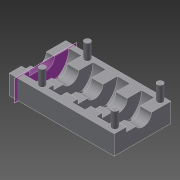
# Autodesk Inventor part: lock housing front
Saved by Autodesk Inventor 2017 (Build 210142000, 142)
## iProperties
Created: 2018-04-20
Part Number: lock housing front
Material: Generic
Document SubType Name: Modeling
Designer: natha
Density: 1 g/cm^3
Appearance: Default
Author: natha
Autodesk Inventor part; units mm, degrees
ref_plane "YZ Plane" through (0, 0, 0) normal (1, 0, 0) x (0, 1, 0)
ref_plane "XZ Plane" through (0, 0, 0) normal (0, 1, 0) x (-1, 0, 0)
sketch "Sketch1" plane through (0, 0, 0) normal (0, 0, 1) x (1, 0, 0)
  arc A0 (-18.2373, -76.3503) -> (26.9537, -71.5105) centre (0, -33.2365) ccw projected
  line L0 (26.9537, -71.5105) -> (46.8123, -71.5105) projected
  line L1 (46.8123, -71.5105) -> (46.8123, -74.3095) projected
  arc A1 (23.0377, -99.6575) -> (46.8123, -74.3095) centre (21.4123, -74.3095) ccw projected
  line L2 (23.0377, -99.6575) -> (23.0377, -92.0895) projected
  line L3 (23.0377, -92.0895) -> (-18.2373, -92.0895) projected
  line L4 (-18.2373, -76.3503) -> (-18.2373, -92.0895) projected
  arc A2 (21.4123, -99.7095) -> (46.8123, -74.3095) centre (21.4123, -74.3095) ccw projected
  line L5 (46.8123, -74.3095) -> (46.8123, -71.5105) projected
  line L6 (46.8123, -71.5105) -> (26.9537, -71.5105) projected
  arc A3 (-26.9537, -71.5105) -> (26.9537, -71.5105) centre (0, -33.2365) ccw projected
  line L7 (-26.9537, -71.5105) -> (-46.8123, -71.5105) projected
  line L8 (-46.8123, -71.5105) -> (-46.8123, -74.3095) projected
  arc A4 (-46.8123, -74.3095) -> (-21.4123, -99.7095) centre (-21.4123, -74.3095) ccw projected
  line L9 (-21.4123, -99.7095) -> (21.4123, -99.7095) projected
  line L10 (-18.2373, -92.0895) -> (-18.2373, -99.7095)
  line L11 (-18.2373, -92.0895) -> (23.0377, -92.0895)
  line L12 (23.0377, -92.0895) -> (23.0377, -99.6575)
  point P0 (0, 0)
  constraints: 6 end point, 2 collinear, 1 perpendicular, 1 point on line
ref_plane "Work Plane1" through (-46.8123, -99.7095, 22.225) normal (0, 0, -1) x (0, 1, 0)
extrude "Extrusion1" add sketch "Sketch1" along normal up to surface (22.225 mm away) contours L3 L2 A2 L9 L10
sketch "Sketch2" plane through (-18.2373, -92.0895, 22.225) normal (0, 1, 0) x (1, 0, 0)
  circle A0 centre (39.0525, 2.4765) radius 1.27 projected
  circle A1 centre (39.0525, 20.2565) radius 1.27 projected
  circle A2 centre (10.4775, 20.2565) radius 1.27 projected
  circle A3 centre (10.4775, 2.4765) radius 1.27 projected
  circle A4 centre (39.0525, 2.4765) radius 1.143
  circle A5 centre (39.0525, 20.2565) radius 1.143
  circle A6 centre (10.4775, 2.4765) radius 1.143
  circle A7 centre (10.4775, 20.2565) radius 1.143
  point P0 (18.2373, 22.225)
  dimension "d4" = 0.127
  dimension "d5" = 0.127
  dimension "d6" = 0.127
  dimension "d7" = 0.127
  constraints: 4 centre point
  measures "d4" radial gap between concentric circles of A0 A4
  measures "d5" radial gap between concentric circles of A1 A5
  measures "d6" radial gap between concentric circles of A3 A6
  measures "d7" radial gap between concentric circles of A2 A7
extrude "Extrusion2" add sketch "Sketch2" along normal blind 6.096 contours A4 | A5 | A6 | A7
ref_plane "Work Plane2" through (-15.0623, -99.7095, 0) normal (-1, 0, 0) x (0, 0, 1)
sketch "Sketch3" plane through (-15.0623, -99.7095, 0) normal (-1, 0, 0) x (0, 0, 1)
  arc A0 (8.8042, -0.8832) -> (13.0521, -0.8802) centre (10.922, 7.62) ccw projected
  circle A1 centre (10.922, 7.62) radius 3.175 projected
  line L0 (13.744, 9.3345) -> (17.399, 9.3345) projected
  line L1 (17.399, 9.3345) -> (17.399, 7.62) projected
  line L2 (17.399, 9.3345) -> (17.399, 5.9055) projected
  line L3 (17.399, 5.9055) -> (13.744, 5.9055) projected
  arc A2 (13.744, 9.3345) -> (13.744, 5.9055) centre (10.922, 7.62) ccw projected
  arc A3 (19.7485, 7.62) -> (1.9685, 7.62) centre (10.8585, 7.62) ccw projected
  arc A4 (1.9685, 7.62) -> (19.7485, 7.62) centre (10.8585, 7.62) ccw
  line L4 (19.7485, 7.62) -> (17.399, 7.62)
  line L5 (18.6055, 7.62) -> (20.8915, 7.62) projected
  line L6 (0, 7.62) -> (22.225, 7.62) projected
  line L7 (7.62, 7.62) -> (1.9685, 7.62)
  point P0 (0, 99.7095)
  constraints: 4 end point, 3 point on circle, 2 collinear, 1 centre point, 1 coincident, 1 point on line
extrude "Extrusion3" cut sketch "Sketch3" against normal blind 5.08
pattern_linear "Rectangular Pattern1" count 4 spacing 9.525 along (1, 0, 0) of "Extrusion3"
sketch "Sketch4" plane through (-18.2373, -99.7095, 0) normal (-1, 0, 0) x (0, 0, 1)
  line L0 (17.399, 9.3345) -> (17.399, 5.9055) projected
  line L1 (17.399, 5.9055) -> (13.744, 5.9055) projected
  arc A0 (13.744, 9.3345) -> (13.744, 5.9055) centre (10.922, 7.62) ccw projected
  line L2 (1.9685, 7.62) -> (19.7485, 7.62) projected
  line L3 (17.399, 7.62) -> (7.62, 7.62)
  point P0 (0, 99.7095)
  constraints: 2 end point, 2 point on line, 1 midpoint, 1 point on circle
extrude "Extrusion4" cut sketch "Sketch4" against normal through all
body "Solid1"
